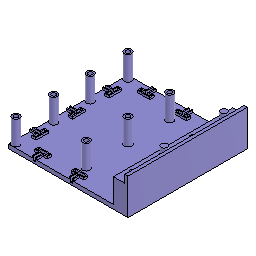
Masa Teren Dreapta (Autodesk Fusion 360 design; units mm, degrees)
part number: 2026-06-02-22-20-48-873
Autodesk Fusion 360 part; units mm, degrees
note: some values were not read from the file. Chosen so that the rebuilt part matches the saved one: which bodies a step acts on.
sketch "Sketch1" plane through (0, 0, 0) normal (0, 0, 1) x (1, 0, 0)
  line L0 (-67.5, 42.5803) -> (46.8447, 42.5803)
  line L1 (-5.5, 36.5803) -> (-5.5, 42.5803)
  line L2 (-9.5, 42.5803) -> (-9.5, 36.5803)
  line L3 (-1.5, 36.5803) -> (-5.5, 36.5803)
  line L4 (-1.5, 32.5803) -> (-1.5, 36.5803)
  line L5 (-13.5, 32.5803) -> (-1.5, 32.5803)
  line L6 (-13.5, 36.5803) -> (-13.5, 32.5803)
  line L7 (-9.5, 36.5803) -> (-13.5, 36.5803)
  line L8 (-40.5, 36.5803) -> (-40.5, 42.5803)
  line L9 (-44.5, 42.5803) -> (-44.5, 36.5803)
  line L10 (-36.5, 36.5803) -> (-40.5, 36.5803)
  line L11 (-36.5, 32.5803) -> (-36.5, 36.5803)
  line L12 (-48.5, 32.5803) -> (-36.5, 32.5803)
  line L13 (-48.5, 36.5803) -> (-48.5, 32.5803)
  line L14 (-44.5, 36.5803) -> (-48.5, 36.5803)
  line L15 (46.8447, 42.5803) -> (46.8447, 156.9249)
  line L16 (46.8447, 156.9249) -> (-67.5, 156.9249)
  line L17 (-67.5, 156.9249) -> (-67.5, 42.5803)
  line L18 (-5.5, 42.5803) -> (-5.5, 48.5803)
  line L19 (-5.5, 48.5803) -> (-1.5, 48.5803)
  line L20 (-1.5, 48.5803) -> (-1.5, 52.5803)
  line L21 (-1.5, 52.5803) -> (-13.5, 52.5803)
  line L22 (-13.5, 52.5803) -> (-13.5, 48.5803)
  line L23 (-13.5, 48.5803) -> (-9.5, 48.5803)
  line L24 (-9.5, 48.5803) -> (-9.5, 42.5803)
  line L25 (-6.5, 42.5803) -> (-6.5, 49.5803)
  line L26 (-6.5, 49.5803) -> (-2.5, 49.5803)
  line L27 (-2.5, 49.5803) -> (-2.5, 51.5803)
  line L28 (-2.5, 51.5803) -> (-12.5, 51.5803)
  line L29 (-12.5, 51.5803) -> (-12.5, 49.5803)
  line L30 (-12.5, 49.5803) -> (-8.5, 49.5803)
  line L31 (-8.5, 49.5803) -> (-8.5, 42.5803)
  line L32 (-40.5, 42.5803) -> (-40.5, 48.5803)
  line L33 (-44.5, 42.5803) -> (-44.5, 48.5803)
  line L34 (-44.5, 48.5803) -> (-48.5, 48.5803)
  line L35 (-48.5, 48.5803) -> (-48.5, 52.5803)
  line L36 (-48.5, 52.5803) -> (-36.5, 52.5803)
  line L37 (-36.5, 52.5803) -> (-36.5, 48.5803)
  line L38 (-36.5, 48.5803) -> (-40.5, 48.5803)
  line L39 (-43.5, 42.5803) -> (-43.5, 49.5803)
  line L40 (-43.5, 49.5803) -> (-47.5, 49.5803)
  line L41 (-47.5, 49.5803) -> (-47.5, 51.5803)
  line L42 (-47.5, 51.5803) -> (-37.5, 51.5803)
  line L43 (-37.5, 51.5803) -> (-37.5, 49.5803)
  line L44 (-37.5, 49.5803) -> (-41.5, 49.5803)
  line L45 (-41.5, 42.5803) -> (-41.5, 49.5803)
  line L46 (46.8447, 99.7526) -> (-67.5, 99.7526) construction
  line L47 (-5.5, 156.9249) -> (-5.5, 150.9249)
  line L48 (-5.5, 150.9249) -> (-1.5, 150.9249)
  line L49 (-1.5, 150.9249) -> (-1.5, 146.9249)
  line L50 (-1.5, 146.9249) -> (-13.5, 146.9249)
  line L51 (-2.5, 147.9249) -> (-12.5, 147.9249)
  line L52 (-12.5, 149.9249) -> (-8.5, 149.9249)
  line L53 (-12.5, 147.9249) -> (-12.5, 149.9249)
  line L54 (-6.5, 156.9249) -> (-6.5, 149.9249)
  line L55 (-6.5, 149.9249) -> (-2.5, 149.9249)
  line L56 (-2.5, 149.9249) -> (-2.5, 147.9249)
  line L57 (-8.5, 149.9249) -> (-8.5, 156.9249)
  line L58 (-9.5, 150.9249) -> (-9.5, 156.9249)
  line L59 (-13.5, 150.9249) -> (-9.5, 150.9249)
  line L60 (-13.5, 146.9249) -> (-13.5, 150.9249)
  line L61 (-48.5, 146.9249) -> (-36.5, 146.9249)
  line L62 (-48.5, 150.9249) -> (-48.5, 146.9249)
  line L63 (-44.5, 150.9249) -> (-48.5, 150.9249)
  line L64 (-43.5, 149.9249) -> (-47.5, 149.9249)
  line L65 (-47.5, 149.9249) -> (-47.5, 147.9249)
  line L66 (-47.5, 147.9249) -> (-37.5, 147.9249)
  line L67 (-37.5, 147.9249) -> (-37.5, 149.9249)
  line L68 (-36.5, 146.9249) -> (-36.5, 150.9249)
  line L69 (-36.5, 150.9249) -> (-40.5, 150.9249)
  line L70 (-40.5, 156.9249) -> (-40.5, 150.9249)
  line L71 (-41.5, 156.9249) -> (-41.5, 149.9249)
  line L72 (-37.5, 149.9249) -> (-41.5, 149.9249)
  line L73 (-43.5, 156.9249) -> (-43.5, 149.9249)
  line L74 (-44.5, 156.9249) -> (-44.5, 150.9249)
  line L75 (30.5, 149.9249) -> (30.5, 147.9249)
  line L76 (31.5, 146.9249) -> (19.5, 146.9249)
  line L77 (19.5, 150.9249) -> (23.5, 150.9249)
  line L78 (30.5, 147.9249) -> (20.5, 147.9249)
  line L79 (26.5, 149.9249) -> (30.5, 149.9249)
  line L80 (31.5, 150.9249) -> (31.5, 146.9249)
  line L81 (20.5, 147.9249) -> (20.5, 149.9249)
  line L82 (27.5, 150.9249) -> (31.5, 150.9249)
  line L83 (20.5, 149.9249) -> (24.5, 149.9249)
  line L84 (19.5, 146.9249) -> (19.5, 150.9249)
  line L85 (26.5, 156.9249) -> (26.5, 149.9249)
  line L86 (27.5, 156.9249) -> (27.5, 150.9249)
  line L87 (24.5, 149.9249) -> (24.5, 156.9249)
  line L88 (23.5, 150.9249) -> (23.5, 156.9249)
  line L89 (-67.5, 101.7526) -> (-61.5, 101.7526)
  line L90 (-61.5, 101.7526) -> (-61.5, 105.7526)
  line L91 (-61.5, 105.7526) -> (-57.5, 105.7526)
  line L92 (-57.5, 105.7526) -> (-57.5, 93.7526)
  line L93 (-57.5, 93.7526) -> (-61.5, 93.7526)
  line L94 (-61.5, 93.7526) -> (-61.5, 97.7526)
  line L95 (-61.5, 97.7526) -> (-67.5, 97.7526)
  line L96 (-67.5, 100.7526) -> (-60.5, 100.7526)
  line L97 (-60.5, 100.7526) -> (-60.5, 104.7526)
  line L98 (-60.5, 104.7526) -> (-58.5, 104.7526)
  line L99 (-58.5, 104.7526) -> (-58.5, 94.7526)
  line L100 (-58.5, 94.7526) -> (-60.5, 94.7526)
  line L101 (-60.5, 94.7526) -> (-60.5, 98.7526)
  line L102 (-60.5, 98.7526) -> (-67.5, 98.7526)
  line L103 (-67.5, 65.7526) -> (-60.5, 65.7526)
  line L104 (-60.5, 65.7526) -> (-60.5, 69.7526)
  line L105 (-60.5, 69.7526) -> (-58.5, 69.7526)
  line L106 (-58.5, 69.7526) -> (-58.5, 59.7526)
  line L107 (-58.5, 59.7526) -> (-60.5, 59.7526)
  line L108 (-60.5, 59.7526) -> (-60.5, 63.7526)
  line L109 (-60.5, 63.7526) -> (-67.5, 63.7526)
  line L110 (-61.5, 66.7526) -> (-61.5, 70.7526)
  line L111 (-61.5, 70.7526) -> (-57.5, 70.7526)
  line L112 (-57.5, 70.7526) -> (-57.5, 58.7526)
  line L113 (-57.5, 58.7526) -> (-61.5, 58.7526)
  line L114 (-61.5, 58.7526) -> (-61.5, 62.7526)
  line L115 (-61.5, 62.7526) -> (-67.5, 62.7526)
  line L116 (-67.5, 66.7526) -> (-61.5, 66.7526)
  line L117 (-67.5, 135.7526) -> (-60.5, 135.7526)
  line L118 (-60.5, 135.7526) -> (-60.5, 139.7526)
  line L119 (-60.5, 139.7526) -> (-58.5, 139.7526)
  line L120 (-58.5, 139.7526) -> (-58.5, 129.7526)
  line L121 (-58.5, 129.7526) -> (-60.5, 129.7526)
  line L122 (-60.5, 129.7526) -> (-60.5, 133.7526)
  line L123 (-60.5, 133.7526) -> (-67.5, 133.7526)
  line L124 (-61.5, 136.7526) -> (-61.5, 140.7526)
  line L125 (-61.5, 140.7526) -> (-57.5, 140.7526)
  line L126 (-57.5, 140.7526) -> (-57.5, 128.7526)
  line L127 (-57.5, 128.7526) -> (-61.5, 128.7526)
  line L128 (-61.5, 128.7526) -> (-61.5, 132.7526)
  line L129 (-61.5, 132.7526) -> (-67.5, 132.7526)
  line L130 (-67.5, 136.7526) -> (-61.5, 136.7526)
  line L131 (-10.3277, 156.9249) -> (-10.3277, 42.5803) construction
  circle A0 centre (-10.3277, 99.7526) radius 3.5
  circle A1 centre (-10.3277, 99.7526) radius 2
  line L132 (32.8447, 42.5803) -> (32.8447, 156.9249)
  line L133 (43.8447, 42.5803) -> (43.8447, 156.9249)
  circle A2 centre (38.3447, 56.5803) radius 5.5
  line L134 (43.8447, 42.5803) -> (32.8447, 42.5803)
  circle A3 centre (38.3447, 56.5803) radius 3
  circle A4 centre (38.3447, 85.7526) radius 5.5
  circle A5 centre (38.3447, 85.7526) radius 3
  circle A6 centre (38.3447, 113.7526) radius 5.5
  circle A7 centre (38.3447, 113.7526) radius 3
  circle A8 centre (38.3447, 142.9249) radius 5.5
  circle A9 centre (38.3447, 142.9249) radius 3
  circle A10 centre (-64, 153.4249) radius 3.5
  circle A11 centre (-64, 153.4249) radius 2
  circle A12 centre (-64, 46.0803) radius 3.5
  circle A13 centre (-64, 46.0803) radius 2
  circle A14 centre (-64, 117.2526) radius 3.5
  circle A15 centre (-64, 117.2526) radius 2
  circle A16 centre (-64, 82.2526) radius 3.5
  circle A17 centre (-64, 82.2526) radius 2
  circle A18 centre (-10.3277, 59.7526) radius 3.5
  circle A19 centre (-10.3277, 59.7526) radius 2
  circle A20 centre (-10.3277, 139.7526) radius 3.5
  circle A21 centre (-10.3277, 139.7526) radius 2
  point P0 (-10.3277, 156.9249)
  dimension "d605" = 114.3447
  dimension "d606" = 114.3447
  dimension "d607" = 32.5803
  dimension "d608" = 1.5
  dimension "d609" = 10
  dimension "d610" = 48.3447
  dimension "d611" = 35
  dimension "d612" = 12
  dimension "d613" = 4
  dimension "d614" = 43
  dimension "d615" = 6
  dimension "d616" = 4
  dimension "d617" = 4
  dimension "d618" = 12
  dimension "d619" = 4
  dimension "d620" = 4
  dimension "d621" = -1
  dimension "d622" = 6
  dimension "d623" = 6
  dimension "d624" = 4
  dimension "d625" = 4
  dimension "d626" = 12
  dimension "d627" = 4
  dimension "d628" = 1
  dimension "d631" = 33
  dimension "d632" = 0
  dimension "d633" = 21
  dimension "d634" = 23
  dimension "d635" = 19
  dimension "d636" = 15.3447
  dimension "d637" = 6
  dimension "d638" = 4
  dimension "d639" = 4
  dimension "d640" = 12
  dimension "d641" = 2
  dimension "d642" = 4
  dimension "d643" = 4
  dimension "d644" = 1
  dimension "d647" = 0
  dimension "d648" = 35
  dimension "d649" = 7
  dimension "d650" = 4
  dimension "d651" = 14
  dimension "d652" = 3
  dimension "d653" = 14
  dimension "d654" = 6
  dimension "d655" = 14
  dimension "d656" = 6
  dimension "d657" = 3.5
  dimension "d658" = 4
  dimension "d659" = 3.5
  dimension "d660" = 4
  dimension "d661" = 31
  dimension "d662" = 7
  dimension "d663" = 15.5
  dimension "d664" = 4
  dimension "d667" = 0
  dimension "d668" = 40
  constraint perpendicular L0 L15
  constraint perpendicular L15 L16
  constraint perpendicular L0 L17
  constraint coincident L0 L2.start
  constraint coincident L0 L1.end
  constraint perpendicular L4 L5
  constraint perpendicular L5 L6
  constraint perpendicular L6 L7
  constraint perpendicular L2 L7
  constraint perpendicular L3 L4
  constraint perpendicular L1 L3
  constraint collinear L5 L12
  constraint collinear L3 L7
  constraint collinear L7 L10
  constraint vertical L4
  constraint horizontal L0.start L2.start
  constraint horizontal L2.start L9.start
  constraint equal L5 L12
  constraint equal L3 L6
  constraint equal L3 L7
  constraint equal L3 L10
  constraint equal L3 L13
  constraint equal L3 L14
  constraint equal L1 L8
  constraint equal L1 L9
  constraint perpendicular L8 L10
  constraint perpendicular L0 L18
  constraint perpendicular L18 L19
  constraint perpendicular L19 L20
  constraint perpendicular L20 L21
  constraint perpendicular L21 L22
  constraint perpendicular L22 L23
  constraint perpendicular L0 L32
  constraint perpendicular L0 L33
  constraint perpendicular L33 L34
  constraint perpendicular L34 L35
  constraint perpendicular L35 L36
  constraint perpendicular L36 L37
  constraint midpoint L15 L46.start
  constraint midpoint L17 L46.end
  constraint symmetric L1.end L46 L47.start
  constraint symmetric L2.start L46 L58.end
  constraint symmetric L8.end L46 L70.start
  constraint symmetric L9.start L46 L74.start
  constraint symmetric L18.end L46 L47.end
  constraint symmetric L19.end L46 L48.end
  constraint symmetric L20.end L46 L49.end
  constraint symmetric L21.end L46 L50.end
  constraint symmetric L22.end L46 L59.start
  constraint symmetric L23.end L46 L58.start
  constraint symmetric L25.start L46 L54.start
  constraint symmetric L25.end L46 L54.end
  constraint symmetric L26.end L46 L55.end
  constraint symmetric L27.end L46 L51.start
  constraint symmetric L28.end L46 L51.end
  constraint symmetric L29.end L46 L52.start
  constraint symmetric L30.end L46 L52.end
  constraint symmetric L31.end L46 L57.end
  constraint symmetric L32.end L46 L69.end
  constraint symmetric L33.end L46 L63.start
  constraint symmetric L34.end L46 L62.start
  constraint symmetric L35.end L46 L61.start
  constraint symmetric L36.end L46 L61.end
  constraint symmetric L37.end L46 L68.end
  constraint symmetric L39.start L46 L73.start
  constraint symmetric L39.end L46 L64.start
  constraint symmetric L40.end L46 L64.end
  constraint symmetric L41.end L46 L65.end
  constraint symmetric L42.end L46 L66.end
  constraint symmetric L43.end L46 L67.end
  constraint symmetric L44.end L46 L71.end
  constraint symmetric L45.start L46 L71.start
  constraint coincident L17 L89.start
  constraint perpendicular L17 L89
  constraint perpendicular L89 L90
  constraint perpendicular L90 L91
  constraint perpendicular L91 L92
  constraint perpendicular L92 L93
  constraint perpendicular L93 L94
  constraint coincident L17 L95.end
  constraint perpendicular L17 L95
  constraint coincident L16 P0
  constraint midpoint L16 P0
  constraint coincident P0 L131.start
  constraint midpoint L0 L131.end
  constraint midpoint L131 A0.centre
  constraint concentric A0 A1
  constraint coincident L0 L132.start
  constraint coincident L16 L132.end
  constraint perpendicular L16 L132
  constraint coincident L0 L133.start
  constraint coincident L16 L133.end
  constraint perpendicular L16 L133
  constraint tangent L133 A2
  constraint tangent L132 A2
  constraint concentric A2 A3
  constraint tangent L132 A4
  constraint tangent L133 A4
  constraint concentric A4 A5
  constraint symmetric L46 A2 A8
  constraint symmetric L46 A3 A9
  constraint symmetric L46 A4 A6
  constraint symmetric L46 A5 A7
  constraint tangent L16 A10
  constraint tangent L17 A10
  constraint concentric A10 A11
  constraint tangent L0 A12
  constraint tangent L17 A12
  constraint concentric A12 A13
  constraint concentric A14 A15
  constraint tangent L17 A14
  constraint symmetric L46 A14 A16
  constraint symmetric L46 A15 A17
  measures "d605" distance of L0.end L15.end
  measures "d606" distance of L0.start L0.end
  measures "d607" distance of origin L5
  measures "d608" distance of origin L4
  measures "d609" distance of L0 L5
  measures "d610" distance of L4 L15
  measures "d611" distance of L4 L11
  measures "d612" distance of L4 L6
  measures "d613" distance of L3 L5
  measures "d614" distance of L4 L9
  measures "d615" distance of L1.end L18.end
  measures "d616" distance of L18.end L19.end
  measures "d617" distance of L19.end L20.end
  measures "d618" distance of L20.end L21.end
  measures "d619" distance of L21.end L22.end
  measures "d620" distance of L22.end L23.end
  measures "d622" distance of L8.end L32.end
  measures "d623" distance of L9.start L33.end
  measures "d624" distance of L33.end L34.end
  measures "d625" distance of L34.end L35.end
  measures "d626" distance of L35.end L36.end
  measures "d627" distance of L36.end L37.end
  measures "d633" distance of L49 L84
  measures "d634" distance of L60 L68
  measures "d635" distance of L17 L62
  measures "d636" distance of L15 L80
  measures "d637" distance of L89.start L89.end
  measures "d638" distance of L89.end L90.end
  measures "d639" distance of L90.end L91.end
  measures "d640" distance of L91.end L92.end
  measures "d641" distance of L46 L89
  measures "d642" distance of L92.end L93.end
  measures "d643" distance of L93.end L94.end
  measures "d649" diameter of A0
  measures "d650" diameter of A1
  measures "d651" distance of L15 L132
  measures "d652" distance of L15 L133
  measures "d653" distance of A2.centre L134
  measures "d654" diameter of A3
  measures "d655" distance of L46 A4.centre
  measures "d656" diameter of A5
  measures "d657" radius of A10
  measures "d658" diameter of A11
  measures "d659" radius of A12
  measures "d660" diameter of A13
  measures "d661" distance of L89 L129
  measures "d662" diameter of A14
  measures "d663" distance of L129 A14.centre
  measures "d664" diameter of A15
extrude "Extrude1" add sketch "Sketch1" along normal blind 4 contours L0 L16 L17 L18 L19 L20 L21 L22 L23 L24 L32 L33 L34 L35 L36 L37 L38 L47 L48 L49 L50 L58 L59 L60 L61 L62 L63 L68 L69 L70 L74 L76 L77 L80 L82 L84 L86 L88 L89 L90 L91 L92 L93 L94 L95 L110 L111 L112 L113 L114 L115 L116 L124 L125 L126 L127 L128 L129 L130 L132 A10 A12 | L0 L17 A12 | L16 L17 A10 makes body 1 at (19.1593, 96.2454, 0)
extrude "Extrude2" add sketch "Sketch1" along normal blind 34.5 separate body contours L0 L15 L16 L133 makes body 2
extrude "Extrude3" add sketch "Sketch1" along normal blind 27 contours L0 L132 L133 A2 L134 | L132 L133 A2 A4 | A2 | L132 L133 A4 A6 | A4 | L132 L133 A6 A8 | A6 | L16 L132 L133 A8 | A8 bodies 1 2
extrude "Extrude4" add sketch "Sketch1" along normal blind 22 separate body contours A3 | A7 makes body 3 at (41.341, 56.4307, 14.6667) makes body 4 at (35.5803, 112.5873, 14.6667)
extrude "Extrude5" add sketch "Sketch1" along normal blind 34 separate body contours A5 | A9 makes body 5 at (40.9794, 87.1874, 22.6667) makes body 6 at (41.1638, 143.951, 11.3333)
extrude "Extrude6" add sketch "Sketch1" along normal blind 6 separate body contours L0 L32 L33 L34 L35 L36 L37 L38 L39 L40 L41 L42 L43 L44 L45 | L17 L103 L104 L105 L106 L107 L108 L109 L110 L111 L112 L113 L114 L115 L116 | L0 L18 L19 L20 L21 L22 L23 L24 L25 L26 L27 L28 L29 L30 L31 | L17 L89 L90 L91 L92 L93 L94 L95 L96 L97 L98 L99 L100 L101 L102 | L17 L117 L118 L119 L120 L121 L122 L123 L124 L125 L126 L127 L128 L129 L130 | L16 L75 L76 L77 L78 L79 L80 L81 L82 L83 L84 L85 L86 L87 L88 | L16 L47 L48 L49 L50 L51 L52 L53 L54 L55 L56 L57 L58 L59 L60 | L16 L61 L62 L63 L64 L65 L66 L67 L68 L69 L70 L71 L72 L73 L74 makes body 7 at (-44.5, 146.9249, 2) makes body 8 at (-44.5, 52.5803, 2) makes body 9 at (-57.5, 66.7526, 2) makes body 10 at (-5.5, 146.9249, 2) makes body 11 at (-57.5, 136.7526, 2) makes body 12 at (-5.5, 52.5803, 2) makes body 13 at (-57.5, 101.7526, 2) makes body 14 at (27.5, 146.9249, 2)
extrude "Extrude7" add sketch "Sketch1" along normal blind 2 contours L0 L39 L40 L41 L42 L43 L44 L45 | L17 L103 L104 L105 L106 L107 L108 L109 | L0 L25 L26 L27 L28 L29 L30 L31 | L17 L96 L97 L98 L99 L100 L101 L102 | L17 L117 L118 L119 L120 L121 L122 L123 | L16 L75 L78 L79 L81 L83 L85 L87 | L16 L51 L52 L53 L54 L55 L56 L57 | L16 L64 L65 L66 L67 L71 L72 L73 bodies 7 8 9 10 11 12 13 14
extrude "Extrude8" add sketch "Sketch1" along normal blind 27 contours A14 | A16 | A12 | A10 | A0 | A18 | A20 bodies 1
extrude "Extrude9" add sketch "Sketch1" along normal blind 22 contours A1 | A11 | A13 | A15 | A17 | A19 | A21 bodies 1
combine "Combine1" operation add target body 1 tool bodies 6 9 11 13 3 4 5 7 8 10 12 14
equation "d605 = d606"
equation "d663 = d661 / 2"
named bodies: "Poarta Dreapta Sus"
